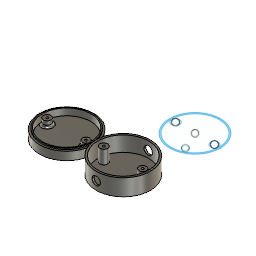
Sonoff Slampher v2 (Autodesk Fusion 360 design; units mm, degrees)
Autodesk Fusion 360 part; units mm, degrees
sketch "Esquisse1" plane through (0, 0, 0) normal (0, 0, 1) x (1, 0, 0)
  circle A0 centre (39.418507, -39.626419) radius 33.5
  circle A1 centre (39.418507, -39.626419) radius 32
  circle A2 centre (65.168507, -39.626419) radius 4.926122
  circle A3 centre (13.668507, -39.626419) radius 5.131771
  circle A4 centre (49.926466, -62.944442) radius 3.5
  circle A5 centre (13.668507, -39.626419) radius 1
  circle A6 centre (65.168507, -39.626419) radius 1
  dimension "d8" = 2
  dimension "d9" = 2
  constraint concentric A3 A5
  constraint concentric A2 A6
  measures "d8" diameter of A5
  measures "d9" diameter of A6
extrude "Extrusion1" add sketch "Esquisse1" along normal blind 2 contours A0 | A1 picked at (70.342665, -50.906942) picked at (40.281132, -28.001373) makes body 1
extrude "Extrusion2" add sketch "Esquisse1" along normal blind 20 thin wall 1.5 on the left open curves A0 bodies 1
extrude "Extrusion3" add sketch "Esquisse1" along normal blind 2 contours A2 | A3 | A4 | A5 | A6 picked at (68.767581, -39.871152) picked at (17.403915, -39.881369) picked at (49.666858, -61.909819) picked at (13.923944, -40.001075) picked at (65.487031, -40.178119) bodies 1
extrude "Extrusion4" add sketch "Esquisse1" along normal blind 20 contours A2 | A3 picked at (68.767581, -39.871152) picked at (17.403915, -39.881369) bodies 1
extrude "Extrusion5" add 1 faces at (73.7882, -41.365245, 20) along direction (0, 0, 1) blind 2 on bodies 1 bodies 1
extrude "Extrusion6" cut sketch "Esquisse1" along normal blind 3 contours A4 picked at (49.666858, -61.909819) bodies 1
move_body "Déplacer1" bodies 1 to x (1, 0, 0) y (0, 1, 0) z (0, 0, 1) at (0, -95, 0)
extrude "Extrusion7" add sketch "Esquisse1" along normal blind 2 separate body contours A0 | A1 picked at (70.342665, -50.906942) picked at (40.281132, -28.001373) makes body 2
extrude "Extrusion8" add sketch "Esquisse1" along normal blind 10 thin wall 1.5 on the left open curves A0 bodies 2
extrude "Extrusion9" add sketch "Esquisse1" along normal blind 11.5 thin wall 1.5 on the left open curves A1 bodies 2
extrude "Extrusion10" add sketch "Esquisse1" along normal blind 2 contours A4 picked at (49.666858, -61.909819) bodies 2
extrude "Extrusion11" add sketch "Esquisse1" along normal blind 10 contours A2 | A3 picked at (68.767581, -39.871152) picked at (17.403915, -39.881369) bodies 2
extrude "Extrusion12" cut sketch "Esquisse1" along normal blind 2 contours A2 | A3 picked at (68.767581, -39.871152) picked at (17.403915, -39.881369) bodies 2
extrude "Extrusion13" add 1 faces at (40.281132, -51.251464, 2) along direction (0, 0, 1) blind 0.5 on bodies 2 bodies 2
sketch "Esquisse2" plane through (0, 0, 0) normal (0, 1, 0) x (1, 0, 0)
  line L0 (4.500031, -21.90314) -> (74.000001, 0)
  line L1 (74.000001, 0) -> (74.000001, -21.90314)
  line L2 (74.000001, -21.90314) -> (4.500031, 0)
  circle A0 centre (39.250016, -10.95157) radius 5.5
  dimension "d34" = 11
  constraint vertical L1
  measures "d34" diameter of A0
move_body "Déplacer2" bodies 2 to x (1, 0, 0) y (0, 1, 0) z (0, 0, 1) at (-80, -90, 0)
extrude "Extrusion14" cut sketch "Esquisse2" against normal blind 200 contours L0 L2 A0 | L0 L2 A0 | L0 L2 A0 | L0 L2 A0 picked at (35.617439, -10.505741) picked at (42.646041, -12.306966) picked at (39.792396, -7.335508) picked at (42.794061, -11.873206) bodies 1
sketch "Esquisse3" plane through (0, 0, 20) normal (0, 0, 1) x (-1, 0, 0)
  circle A0 centre (-13.668507, 134.626419) radius 1
  circle A1 centre (-13.668507, 134.626419) radius 5.131771
  circle A2 centre (-13.668507, 134.626419) radius 1.5
  dimension "d37" = 3
  constraint concentric A0 A2
  measures "d37" diameter of A2
extrude "Extrusion15" cut sketch "Esquisse3" against normal blind 15 contours A2 picked at (-14.396918, 135.739022) bodies 1
sketch "Esquisse4" plane through (0, 0, 20) normal (0, 0, 1) x (-1, 0, 0)
  circle A0 centre (-65.168507, 134.626419) radius 1
  circle A1 centre (-65.168507, 134.626419) radius 4.926122
  circle A2 centre (-65.168507, 134.626419) radius 1.5
  dimension "d40" = 3
  constraint concentric A0 A2
  measures "d40" diameter of A2
extrude "Extrusion16" cut sketch "Esquisse4" against normal blind 15 contours A2 picked at (-64.00458, 133.983189) bodies 1
sketch "Esquisse5" plane through (0, 0, 10) normal (0, 0, 1) x (-1, 0, 0)
  circle A0 centre (66.331493, 129.626419) radius 1
  circle A1 centre (66.331493, 129.626419) radius 5.131771
  circle A2 centre (66.331493, 129.626419) radius 1.5
  dimension "d43" = 3
  constraint concentric A0 A2
  measures "d43" diameter of A2
sketch "Esquisse6" plane through (0, 0, 10) normal (0, 0, 1) x (-1, 0, 0)
  circle A0 centre (14.831493, 129.626419) radius 1
  circle A1 centre (14.831493, 129.626419) radius 4.926122
  circle A2 centre (14.831493, 129.626419) radius 1.5
  dimension "d44" = 3
  constraint concentric A0 A2
  measures "d44" diameter of A2
extrude "Extrusion17" cut sketch "Esquisse6" sketch "Esquisse5" against normal blind 8 contours A2 picked at (13.945392, 130.618031) of sketch 2 contours A2 picked at (67.622219, 129.306268) bodies 2
extrude "Extrusion18" add 1 faces at (-39.647881, -142.715115, 0) along direction (0, 0, -1) blind 1 on bodies 2 bodies 2
move_face "DécalerLesFaces1" offset 1 1 faces at (49.771995, -101.192823, 10.983857) on bodies 1
move_face "DécalerLesFaces2" offset 1 1 faces at (-75.537985, -131.371025, 6.333333) on bodies 2
fillet "Congé2" radius 2.5 2 edges at (-19.424252, -131.40778, 2.5) (-71.115983, -131.482146, 2.5) on bodies 2
